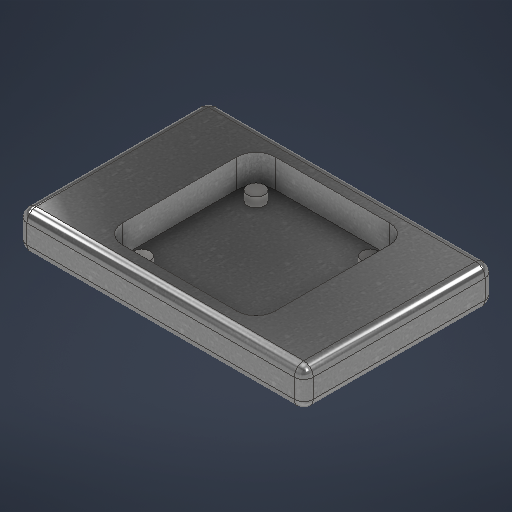
# Autodesk Inventor part: WHEEL_BASE
Saved by Autodesk Inventor 2027.1 (Build 311270010, 270A)
## iProperties
Created: 2026-08-29
Part Number: WHEEL_BASE
Material: Stainless Steel
Document SubType Name: Modeling
Designer: RIDDHIMAN
Density: 8 g/cm^3
Appearance: Semi-Polished
Author: RIDDHIMAN
Autodesk Inventor part; units mm, degrees
ref_plane "YZ Plane" through (0, 0, 0) normal (1, 0, 0) x (0, 1, 0)
ref_plane "XZ Plane" through (0, 0, 0) normal (0, 1, 0) x (-1, 0, 0)
ref_plane "XY Plane" through (0, 0, 0) normal (0, 0, 1) x (1, 0, 0)
sketch "Sketch1" plane through (0, 0, 0) normal (0, 1, 0) x (-1, 0, 0)
  line L0 (375, 250) -> (-375, 250)
  line L1 (-375, 250) -> (-375, -250)
  line L2 (-375, -250) -> (375, -250)
  line L3 (375, -250) -> (375, 250)
  line L4 (375, 250) -> (-375, -250) construction
  line L5 (-375, 250) -> (375, -250) construction
  point P0 (0, 0)
  dimension "d0" = 750
  dimension "d1" = 500
  constraints: 12 end point, 2 midpoint, 2 parallel, 1 horizontal, 1 perpendicular
  measures "d0" distance of L2.end L1.end
  measures "d1" distance of L1.end L0.end
extrude "Extrusion1" add sketch "Sketch1" along normal blind 100
sketch "Sketch2" plane through (0, 100, 0) normal (0, 1, 0) x (1, 0, 0)
  line L0 (-150, -200) -> (150, -200)
  line L1 (200, -150) -> (200, 150)
  line L2 (150, 200) -> (-150, 200)
  line L3 (-200, 150) -> (-200, -150)
  line L4 (-200, -200) -> (200, 200) construction
  line L5 (200, -200) -> (-200, 200) construction
  arc A0 (-200, -150) -> (-150, -200) centre (-150, -150) ccw
  arc A1 (-150, 200) -> (-200, 150) centre (-150, 150) ccw
  arc A2 (150, -200) -> (200, -150) centre (150, -150) ccw
  arc A3 (200, 150) -> (150, 200) centre (150, 150) ccw
  point P0 (0, 0)
  dimension "d4" = 400
  dimension "d5" = 400
  dimension "d6" = 50
  dimension "d7" = 50
  dimension "d8" = 50
  constraints: 12 end point, 8 point on circle, 8 point on line, 8 tangent, 4 centre point, 2 midpoint, 2 parallel, 1 equal radius, 1 horizontal, 1 perpendicular
  measures "d4" distance of L5.end L4.end
  measures "d5" distance of L4.end L5.start
  measures "d6" radius of A0
  measures "d7" radius of A1
  measures "d8" radius of A2
extrude "Extrusion2" cut sketch "Sketch2" against normal blind 75
fillet "Fillet1" radius 25 12 edges at (375, 50, -250) (375, 0, 0) (375, 100, 0) (375, 50, 250) (0, 100, 250) (0, 100, -250) (-375, 100, 0) (0, 0, -250) (-375, 50, -250) (-375, 0, 0) (-375, 50, 250) (0, 0, 250)
sketch "Sketch3" plane through (0, 0, 0) normal (0, -1, 0) x (1, 0, 0)
  line L0 (300, -175) -> (-300, 175) construction
  line L1 (-300, -175) -> (300, 175) construction
  circle A0 centre (-300, -175) radius 25
  circle A1 centre (-300, 175) radius 25
  circle A2 centre (0, -175) radius 25
  circle A3 centre (0, 175) radius 25
  circle A4 centre (300, -175) radius 25
  circle A5 centre (300, 175) radius 25
  point P0 (0, 0)
  dimension "d12" = 600
  dimension "d13" = 350
  dimension "d14" = 50
  dimension "d15" = 50
  dimension "d16" = 50
  dimension "d17" = 50
  dimension "d18" = 50
  dimension "d19" = 50
  constraints: 6 centre point, 4 coincident, 4 end point, 2 midpoint
  measures "d12" distance of L0.end L1.end
  measures "d13" distance of L1.start L0.end
  measures "d14" diameter of A0
  measures "d15" diameter of A1
  measures "d16" diameter of A2
  measures "d17" diameter of A3
  measures "d18" diameter of A4
  measures "d19" diameter of A5
extrude "Extrusion3" cut sketch "Sketch3" against normal blind 10
sketch "Sketch4" plane through (0, 25, 0) normal (0, 1, 0) x (1, 0, 0)
  circle A0 centre (-150, 150) radius 22.5
  arc A1 (-150, 200) -> (-200, 150) centre (-150, 150) ccw projected
  circle A2 centre (150, 150) radius 22.5
  circle A3 centre (150, -150) radius 22.5
  circle A4 centre (-150, -150) radius 22.5
  arc A5 (200, 150) -> (150, 200) centre (150, 150) ccw projected
  arc A6 (150, -200) -> (200, -150) centre (150, -150) ccw projected
  arc A7 (-200, -150) -> (-150, -200) centre (-150, -150) ccw projected
  point P0 (0, 0)
  dimension "d22" = 45
  dimension "d23" = 45
  dimension "d24" = 45
  dimension "d25" = 45
  constraints: 4 centre point, 4 concentric
  measures "d22" diameter of A0
  measures "d23" diameter of A2
  measures "d24" diameter of A3
  measures "d25" diameter of A4
extrude "Extrusion4" add sketch "Sketch4" along normal blind 25
body "Solid1"
